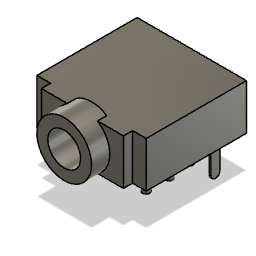
AT-LP60 Headphone Mod 3.5 MM PCB Mount v11 (Autodesk Fusion 360 archive; units mm, degrees)
design "PJ3F07-5P"
Autodesk Fusion 360 part; units mm, degrees
sketch "Sketch1" plane through (0, 0, 0) normal (0, 0, 1) x (1, 0, 0) in component "PJ3F07-5P"
  circle A0 centre (0, 0) radius 1.8
  circle A1 centre (0, 0) radius 3
  dimension "d1" = 3.6
  dimension "d2" = 6
  constraint coincident A0.centre A1.centre
  measures "d1" diameter of A0
  measures "d2" diameter of A1
extrude "Extrude1" add sketch "Sketch1" against normal blind 3 in component "PJ3F07-5P"
ref_plane "WorkPlane1" through (0, 0, -2) normal (0, 0, -1) x (-1, 0, 0) in component "PJ3F07-5P"
sketch "Sketch2" plane through (0, 0, -2) normal (0, 0, -1) x (-1, 0, 0) in component "PJ3F07-5P"
  line L0 (-4.5, 2.5) -> (4.5, 2.5)
  line L1 (4.5, 2.5) -> (4.5, -2.5)
  line L2 (4.5, -2.5) -> (-4.5, -2.5)
  line L3 (-4.5, -2.5) -> (-4.5, 2.5)
  line L4 (-4.5, 2.5) -> (4.5, -2.5) construction
  line L5 (4.5, 2.5) -> (-4.5, -2.5) construction
  circle A0 centre (0, 0) radius 1.8
  circle A1 centre (0, 0) radius 3
  dimension "d6" = 9
  dimension "d7" = 5
  constraint horizontal L0
  constraint perpendicular L0 L1
  constraint parallel L0 L2
  constraint parallel L1 L3
  constraint coincident L4 A0.centre
  constraint coincident L5 A0.centre
  constraint coincident A0.centre A1.centre
  measures "d6" distance of L1.end L2.end
  measures "d7" distance of L0.end L1.end
extrude "Extrude2" add sketch "Sketch2" along normal blind 1 contours L0 L2 L3 A1 | L0 L1 L2 A1 in component "PJ3F07-5P"
sketch "Sketch3" plane through (0, 0, -3) normal (0, 0, -1) x (-1, 0, 0) in component "PJ3F07-5P"
  circle A0 centre (0, 0) radius 1.8
  arc A1 (-1.6583, -2.5) -> (1.6583, -2.5) centre (0, 0) ccw
  line L0 (1.6583, -2.5) -> (4.5, -2.5)
  line L1 (4.5, -2.5) -> (4.5, 2.5)
  line L2 (4.5, 2.5) -> (1.6583, 2.5)
  arc A2 (1.6583, 2.5) -> (-1.6583, 2.5) centre (0, 0) ccw
  line L3 (-1.6583, 2.5) -> (-4.5, 2.5)
  line L4 (-4.5, 2.5) -> (-4.5, -2.5)
  line L5 (-4.5, -2.5) -> (-1.6583, -2.5)
  line L6 (6, 2.5) -> (-6, 2.5)
  line L7 (-6, 2.5) -> (-6, -2.5)
  line L8 (-6, -2.5) -> (6, -2.5)
  line L9 (6, -2.5) -> (6, 2.5)
  line L10 (6, 2.5) -> (-6, -2.5) construction
  line L11 (-6, 2.5) -> (6, -2.5) construction
  dimension "d10" = 12
  dimension "d11" = 5
  constraint horizontal L6
  constraint perpendicular L6 L7
  constraint parallel L6 L8
  constraint parallel L7 L9
  constraint coincident L10 A0.centre
  constraint coincident L11 A0.centre
  constraint coincident A0.centre A1.centre
  measures "d10" distance of L7.end L8.end
  measures "d11" distance of L6.end L7.end
extrude "Extrude3" add sketch "Sketch3" along normal blind 11 contours L0 L1 L2 L3 L4 L5 L6 L8 | L4 L6 L7 L8 | L1 L6 L8 L9 in component "PJ3F07-5P"
sketch "Sketch4" plane through (0, -2.5, 0) normal (0, -1, 0) x (1, 0, 0) in component "PJ3F07-5P"
  line L0 (-1.6583, -2) -> (-4.5, -2)
  line L1 (-4.5, -2) -> (-4.5, -3)
  line L2 (-4.5, -3) -> (-6, -3)
  line L3 (-6, -3) -> (-6, -14)
  line L4 (-6, -14) -> (6, -14)
  line L5 (6, -14) -> (6, -3)
  line L6 (6, -3) -> (4.5, -3)
  line L7 (4.5, -3) -> (4.5, -2)
  line L8 (4.5, -2) -> (1.6583, -2)
  line L9 (1.6583, -2) -> (1.6583, -3)
  line L10 (1.6583, -3) -> (-1.6583, -3)
  line L11 (-1.6583, -3) -> (-1.6583, -2)
  circle A0 centre (5, -4) radius 0.5
  circle A1 centre (5, -6.5) radius 0.5
  circle A2 centre (-5, -4) radius 0.5
  circle A3 centre (-5, -6.5) radius 0.5
  circle A4 centre (0, -11.5) radius 0.5
  line L12 (0.75, -6.9) -> (-0.75, -6.9)
  line L13 (-0.75, -6.9) -> (-0.75, -6.1)
  line L14 (-0.75, -6.1) -> (0.75, -6.1)
  line L15 (0.75, -6.1) -> (0.75, -6.9)
  line L16 (0.75, -6.9) -> (-0.75, -6.1) construction
  line L17 (-0.75, -6.9) -> (0.75, -6.1) construction
  line L18 (-2.9, -12.25) -> (-2.1, -12.25)
  line L19 (-2.1, -12.25) -> (-2.1, -10.75)
  line L20 (-2.1, -10.75) -> (-2.9, -10.75)
  line L21 (-2.9, -10.75) -> (-2.9, -12.25)
  line L22 (-2.9, -12.25) -> (-2.1, -10.75) construction
  line L23 (-2.1, -12.25) -> (-2.9, -10.75) construction
  line L24 (-5.4, -12.25) -> (-4.6, -12.25)
  line L25 (-4.6, -12.25) -> (-4.6, -10.75)
  line L26 (-4.6, -10.75) -> (-5.4, -10.75)
  line L27 (-5.4, -10.75) -> (-5.4, -12.25)
  line L28 (-5.4, -12.25) -> (-4.6, -10.75) construction
  line L29 (-4.6, -12.25) -> (-5.4, -10.75) construction
  line L30 (4.6, -12.25) -> (5.4, -12.25)
  line L31 (5.4, -12.25) -> (5.4, -10.75)
  line L32 (5.4, -10.75) -> (4.6, -10.75)
  line L33 (4.6, -10.75) -> (4.6, -12.25)
  line L34 (4.6, -12.25) -> (5.4, -10.75) construction
  line L35 (5.4, -12.25) -> (4.6, -10.75) construction
  line L36 (2.1, -12.25) -> (2.9, -12.25)
  line L37 (2.9, -12.25) -> (2.9, -10.75)
  line L38 (2.9, -10.75) -> (2.1, -10.75)
  line L39 (2.1, -10.75) -> (2.1, -12.25)
  line L40 (2.1, -12.25) -> (2.9, -10.75) construction
  line L41 (2.9, -12.25) -> (2.1, -10.75) construction
  line L42 (-1.6583, -2) -> (1.6583, -2) construction
  line L43 (0, -2) -> (0, -14) construction
  line L44 (-5, -14) -> (-5, -3) construction
  line L45 (5, -14) -> (5, -3) construction
  line L46 (5.1, -11) -> (4.9, -11)
  line L47 (4.9, -11) -> (4.9, -12)
  line L48 (4.9, -12) -> (5.1, -12)
  line L49 (5.1, -12) -> (5.1, -11)
  line L50 (5.1, -11) -> (4.9, -12) construction
  line L51 (4.9, -11) -> (5.1, -12) construction
  line L52 (2.6, -11) -> (2.4, -11)
  line L53 (2.4, -11) -> (2.4, -12)
  line L54 (2.4, -12) -> (2.6, -12)
  line L55 (2.6, -12) -> (2.6, -11)
  line L56 (2.6, -11) -> (2.4, -12) construction
  line L57 (2.4, -11) -> (2.6, -12) construction
  line L58 (-2.4, -11) -> (-2.6, -11)
  line L59 (-2.6, -11) -> (-2.6, -12)
  line L60 (-2.6, -12) -> (-2.4, -12)
  line L61 (-2.4, -12) -> (-2.4, -11)
  line L62 (-2.4, -11) -> (-2.6, -12) construction
  line L63 (-2.6, -11) -> (-2.4, -12) construction
  line L64 (-4.9, -11) -> (-5.1, -11)
  line L65 (-5.1, -11) -> (-5.1, -12)
  line L66 (-5.1, -12) -> (-4.9, -12)
  line L67 (-4.9, -12) -> (-4.9, -11)
  line L68 (-4.9, -11) -> (-5.1, -12) construction
  line L69 (-5.1, -11) -> (-4.9, -12) construction
  line L70 (0.5, -6.4) -> (-0.5, -6.4)
  line L71 (-0.5, -6.4) -> (-0.5, -6.6)
  line L72 (-0.5, -6.6) -> (0.5, -6.6)
  line L73 (0.5, -6.6) -> (0.5, -6.4)
  line L74 (0.5, -6.4) -> (-0.5, -6.6) construction
  line L75 (-0.5, -6.4) -> (0.5, -6.6) construction
  circle A5 centre (-5, -4) radius 0.4
  circle A6 centre (-5, -6.5) radius 0.4
  circle A7 centre (0, -11.5) radius 0.4
  circle A8 centre (5, -6.5) radius 0.4
  circle A9 centre (5, -4) radius 0.4
  point P0 (0, -6.5)
  point P1 (-2.5, -11.5)
  point P2 (-5, -11.5)
  point P3 (5, -11.5)
  point P4 (2.5, -11.5)
  point P5 (5, -11.5)
  point P6 (2.5, -11.5)
  point P7 (-2.5, -11.5)
  point P8 (-5, -11.5)
  point P9 (0, -6.5)
  dimension "d14" = 1
  dimension "d15" = 1
  dimension "d16" = 1
  dimension "d17" = 1
  dimension "d18" = 1
  dimension "d19" = 1
  dimension "d20" = 0.8
  dimension "d21" = 1.5
  dimension "d23" = 2.5
  dimension "d24" = 4.5
  dimension "d25" = 1
  dimension "d26" = 2.5
  dimension "d27" = 1.5
  dimension "d28" = 0.8
  dimension "d29" = 0.8
  dimension "d30" = 1.5
  dimension "d31" = 1.5
  dimension "d32" = 0.8
  dimension "d33" = 0.8
  dimension "d34" = 1.5
  dimension "d35" = 5
  dimension "d36" = 2.5
  dimension "d37" = 10
  dimension "d38" = 5
  dimension "d39" = 5
  dimension "d40" = 9.5
  dimension "d41" = 9.5
  dimension "d42" = 9.5
  dimension "d43" = 9.5
  dimension "d44" = 1
  dimension "d45" = 1
  dimension "d48" = 0.2
  dimension "d49" = 1
  dimension "d50" = 1
  dimension "d51" = 0.2
  dimension "d52" = 0.2
  dimension "d53" = 1
  dimension "d54" = 0.2
  dimension "d55" = 1
  dimension "d56" = 1
  dimension "d57" = 0.2
  dimension "d58" = 0.8
  dimension "d59" = 0.8
  dimension "d60" = 0.8
  dimension "d61" = 0.8
  dimension "d62" = 0.8
  constraint horizontal L12
  constraint perpendicular L12 L13
  constraint parallel L12 L14
  constraint parallel L13 L15
  constraint coincident L16 P9
  constraint coincident L17 P9
  constraint horizontal L18
  constraint perpendicular L18 L19
  constraint parallel L18 L20
  constraint parallel L19 L21
  constraint coincident L22 P7
  constraint coincident L23 P7
  constraint horizontal L24
  constraint perpendicular L24 L25
  constraint parallel L24 L26
  constraint parallel L25 L27
  constraint coincident L28 P8
  constraint coincident L29 P8
  constraint horizontal L30
  constraint perpendicular L30 L31
  constraint parallel L30 L32
  constraint parallel L31 L33
  constraint coincident L34 P5
  constraint coincident L35 P5
  constraint horizontal L36
  constraint perpendicular L36 L37
  constraint parallel L36 L38
  constraint parallel L37 L39
  constraint coincident L40 P6
  constraint coincident L41 P6
  constraint coincident L0.start L11.end
  constraint coincident L8.end L9.start
  constraint midpoint L42 L43.start
  constraint perpendicular L12 L43
  constraint coincident P9 L43
  constraint coincident A4.centre L43
  constraint coincident L4 L44.start
  constraint coincident L2 L44.end
  constraint perpendicular L2 L44
  constraint coincident L4 L45.start
  constraint coincident L6 L45.end
  constraint perpendicular L6 L45
  constraint coincident A0.centre L45
  constraint coincident A1.centre L45
  constraint coincident A3.centre L44
  constraint coincident A2.centre L44
  constraint horizontal L46
  constraint perpendicular L46 L47
  constraint parallel L46 L48
  constraint parallel L47 L49
  constraint coincident L50 P5
  constraint coincident L51 P5
  constraint coincident P5 P3
  constraint horizontal L52
  constraint perpendicular L52 L53
  constraint parallel L52 L54
  constraint parallel L53 L55
  constraint coincident L56 P6
  constraint coincident L57 P6
  constraint coincident P6 P4
  constraint horizontal L58
  constraint perpendicular L58 L59
  constraint parallel L58 L60
  constraint parallel L59 L61
  constraint coincident L62 P7
  constraint coincident L63 P7
  constraint coincident P7 P1
  constraint horizontal L64
  constraint perpendicular L64 L65
  constraint parallel L64 L66
  constraint parallel L65 L67
  constraint coincident L68 P8
  constraint coincident L69 P8
  constraint coincident P8 P2
  constraint horizontal L70
  constraint perpendicular L70 L71
  constraint parallel L70 L72
  constraint parallel L71 L73
  constraint coincident L74 P9
  constraint coincident L75 P9
  constraint coincident P9 P0
  constraint concentric A2 A5
  constraint concentric A3 A6
  constraint concentric A4 A7
  constraint concentric A1 A8
  constraint concentric A0 A9
  measures "d14" diameter of A0
  measures "d15" diameter of A1
  measures "d16" diameter of A2
  measures "d17" diameter of A3
  measures "d18" diameter of A4
  measures "d19" distance of L6 A0.centre
  measures "d20" distance of L12.end L13.end
  measures "d21" distance of L13.end L14.end
  measures "d23" distance of A0.centre A1.centre
  measures "d24" distance of L8 P9
  measures "d25" distance of L2 A2.centre
  measures "d26" vertical distance of A2.centre A3.centre
  measures "d27" distance of L36.start L38.end
  measures "d28" distance of L36.start L36.end
  measures "d29" distance of L31.end L32.end
  measures "d30" distance of L30.end L31.end
  measures "d31" distance of L18.end L19.end
  measures "d32" distance of L19.end L20.end
  measures "d33" distance of L25.end L26.end
  measures "d34" distance of L24.end L25.end
  measures "d35" horizontal distance of P7 P6
  measures "d36" horizontal distance of A4.centre P6
  measures "d37" horizontal distance of P8 P5
  measures "d38" horizontal distance of A4.centre P5
  measures "d39" vertical distance of A1.centre P5
  measures "d40" distance of L8 P6
  measures "d41" distance of L8 A4.centre
  measures "d42" distance of L0 P7
  measures "d43" distance of L0 P8
  measures "d44" distance of L3 L44
  measures "d45" distance of L5 L45
  measures "d48" distance of L47.end L48.end
  measures "d49" distance of L46.end L47.end
  measures "d50" distance of L52.start L54.end
  measures "d51" distance of L53.end L54.end
  measures "d52" distance of L59.end L60.end
  measures "d53" distance of L58.end L59.end
  measures "d54" distance of L65.end L66.end
  measures "d55" distance of L64.end L65.end
  measures "d56" distance of L71.end L72.end
  measures "d57" distance of L70.end L71.end
  measures "d58" diameter of A5
  measures "d59" diameter of A6
  measures "d60" diameter of A7
  measures "d61" diameter of A8
  measures "d62" diameter of A9
extrude "Extrude5" add sketch "Sketch4" along normal blind 1 contours A5 | A6 | A7 | A8 | A9 in component "PJ3F07-5P"
extrude "Extrude6" add sketch "Sketch4" along normal blind 3.5 contours L46 L47 L48 L49 | L52 L53 L54 L55 | L58 L59 L60 L61 | L64 L65 L66 L67 | L70 L71 L72 L73 in component "PJ3F07-5P"
fillet "Fillet1" radius 0.5 10 edges at (-5, -6, -12) (-5, -6, -11) (-2.5, -6, -12) (-2.5, -6, -11) (2.5, -6, -12) (2.5, -6, -11) (5, -6, -12) (5, -6, -11) (0.5, -6, -6.5) (-0.5, -6, -6.5) in component "PJ3F07-5P"
component "PJ3F07-5P" placed x (1, 0, 0) y (0, 1, 0) z (0, 0, 1) at (0, 0, 0)
named bodies: "PJ3F07-5P"
